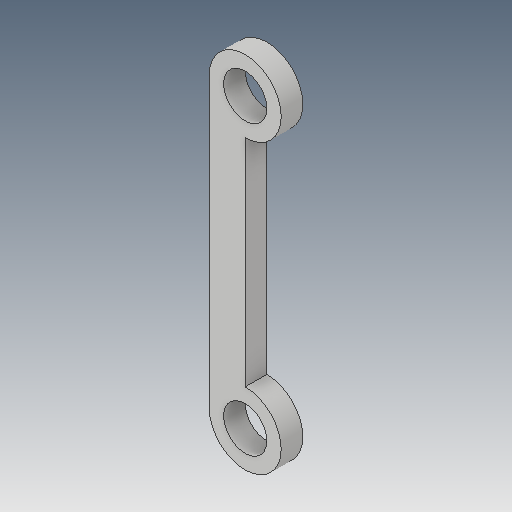
# Autodesk Inventor part: link2
Saved by Autodesk Inventor 2019.4 (Build 234330000, 330)
## iProperties
Created: 2018-08-30
Part Number: link2
Material: 一般
Document SubType Name: Modeling
Designer: AzLIer
Density: 1 g/cm^3
Appearance: 既定
Author: AzLIer
Autodesk Inventor part; units mm, degrees
ref_plane "YZ Plane" through (0, 0, 0) normal (1, 0, 0) x (0, 1, 0)
ref_plane "XZ Plane" through (0, 0, 0) normal (0, 1, 0) x (-1, 0, 0)
ref_plane "XY Plane" through (0, 0, 0) normal (0, 0, 1) x (1, 0, 0)
sketch "スケッチ1" plane through (0, 0, 0) normal (0, 0, 1) x (1, 0, 0)
  circle A0 centre (0, 0) radius 3
  circle A1 centre (0, 40) radius 3
  circle A2 centre (0, 40) radius 5
  circle A3 centre (0, 0) radius 5
  line L0 (0, 5) -> (0, 35)
  line L1 (-5, 40) -> (-5, 0)
  dimension "d0" = 6
  dimension "d1" = 6
  dimension "d2" = 40
  dimension "d3" = 10
  dimension "d4" = 10
  constraints: 4 centre point, 4 end point, 4 point on circle, 2 coincident, 2 tangent, 1 point on line, 1 vertical, 1 vertical alignment
  measures "d0" diameter of A0
  measures "d1" diameter of A1
  measures "d2" distance of point (0, 0) A1.centre
  measures "d3" diameter of A2
  measures "d4" diameter of A3
extrude "押し出し1" add sketch "スケッチ1" along normal blind 3
sketch "スケッチ2" plane through (0, 0, 3) normal (0, 0, 1) x (1, 0, 0)
  circle A0 centre (0, 0) radius 3 projected
  circle A1 centre (0, 40) radius 3 projected
  arc A2 (0, 35) -> (-5, 40) centre (0, 40) ccw projected
  line L0 (-5, 40) -> (-5, 0) projected
  arc A3 (-5, 0) -> (0, 5) centre (0, 0) ccw projected
  line L1 (0, 5) -> (0, 35) projected
  circle A4 centre (0, 0) radius 3
  circle A5 centre (-32.1289, 23.8272) radius 1.25
  line L2 (-4.0161, 2.9784) -> (-5, 3.7081)
  arc A6 (-30.4645, 26.3232) -> (-29.7192, 22.0402) centre (-32.1289, 23.8272) ccw
  line L3 (-5, 9.3436) -> (2.7739, 4.16)
  arc A7 (-4.0161, 2.9784) -> (2.7739, 4.16) centre (0, 0) ccw
  constraints: 4 centre point, 4 end point, 4 point on circle, 2 point on line, 14 other
extrude "押し出し2" [suppressed]
sketch "スケッチ4" plane through (0, 0, 3) normal (0, 0, 1) x (1, 0, 0)
  line L0 (-5, 0) -> (-5, 40) projected
  arc A0 (0, 35) -> (-5, 40) centre (0, 40) ccw projected
  line L1 (0, 35) -> (0, 5) projected
  circle A1 centre (0, 40) radius 3 projected
  circle A2 centre (-27.9404, 11.376) radius 3
  circle A3 centre (0, 40) radius 1.25
  line L2 (-5, 34.8777) -> (-2.0955, 37.8532)
  arc A4 (2.2489, 38.0144) -> (-2.0955, 37.8532) centre (0, 40) ccw
  line L3 (2.2489, 38.0144) -> (-5, 29.8042)
  arc A5 (-24.4479, 14.954) -> (-24.1923, 8.0667) centre (-27.9404, 11.376) ccw
  circle A6 centre (0, 0) radius 3 projected
  arc A7 (-5, 0) -> (0, 5) centre (0, 0) ccw projected
  constraints: 4 end point, 3 centre point, 2 point on circle, 2 point on line, 18 other
extrude "押し出し3" [suppressed]
